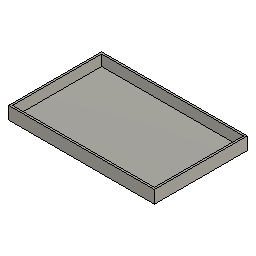
Caja_Tapa (Autodesk Fusion 360 design; units mm, degrees)
Autodesk Fusion 360 part; units mm, degrees
sketch "Sketch1" plane through (0, 0, 0) normal (0, 0, 1) x (1, 0, 0)
  line L0 (0, 0) -> (229, 0)
  line L1 (229, 0) -> (229, 146)
  line L2 (229, 146) -> (0, 146)
  line L3 (0, 146) -> (0, 0)
  dimension "d1" = 229
  dimension "d2" = 146
  constraint horizontal L0
  constraint vertical L1
  constraint horizontal L2
  constraint vertical L3
  constraint coincident L0.start L3.end
  measures "d1" distance of L0.start L0.end
  measures "d2" distance of L0.end L1.end
extrude "Extrude1" add sketch "Sketch1" along normal blind 20
sketch "Sketch2" plane through (0, 0, 20) normal (0, 0, 1) x (-1, 0, 0)
  line L0 (0, -146) -> (0, 0)
  line L1 (0, 0) -> (-229, 0)
  line L2 (-229, 0) -> (-229, -146)
  line L3 (-229, -146) -> (0, -146)
  line L4 (-3, -143) -> (-226, -143)
  line L5 (-226, -143) -> (-226, -3)
  line L6 (-226, -3) -> (-3, -3)
  line L7 (-3, -3) -> (-3, -143)
  dimension "d5" = 3
  dimension "d6" = 3
  dimension "d7" = 3
  dimension "d8" = 3
  constraint horizontal L4
  constraint vertical L5
  constraint horizontal L6
  constraint vertical L7
  measures "d5" distance of L0 L7
  measures "d6" distance of L1 L6
  measures "d7" distance of L3 L4
  measures "d8" distance of L2 L5
extrude "Extrude2" cut sketch "Sketch2" against normal blind 17 contours L4 L5 L6 L7
